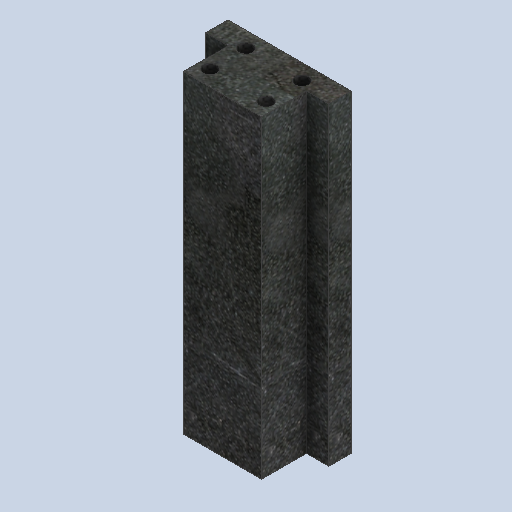
# Autodesk Inventor part: Fuhrung
Saved by Autodesk Inventor 2023.2 (Build 272271000, 271)
## iProperties
Created: 2023-02-07
Part Number: Fuhrung
Material: Steel
Document SubType Name: Modeling
Designer: Ayush
Density: 7.85 g/cm^3
Appearance: Plate
Author: Ayush
Autodesk Inventor part; units mm, degrees
ref_plane "YZ Plane" through (0, 0, 0) normal (1, 0, 0) x (0, 1, 0)
ref_plane "XZ Plane" through (0, 0, 0) normal (0, 1, 0) x (-1, 0, 0)
ref_plane "XY Plane" through (0, 0, 0) normal (0, 0, 1) x (1, 0, 0)
sketch "Sketch1" plane through (0, 0, 0) normal (0, 1, 0) x (-1, 0, 0)
  line L0 (17.5, 0) -> (-17.5, 0)
  line L1 (27.5, -30) -> (-27.5, -30)
  line L2 (27.5, -30) -> (27.5, -20)
  line L3 (27.5, -20) -> (17.5, -20)
  line L4 (-27.5, -30) -> (-27.5, -20)
  line L5 (-27.5, -20) -> (-17.5, -20)
  line L6 (17.5, -20) -> (17.5, 0)
  line L7 (-17.5, -20) -> (-17.5, 0)
  circle A0 centre (12.5, -23) radius 3
  circle A1 centre (-12.5, -23) radius 3
  circle A2 centre (-12.5, -7) radius 3
  circle A3 centre (12.5, -7) radius 3
  point P0 (0, 0)
  dimension "d2" = 35
  dimension "d8" = 55
  dimension "d9" = 10
  dimension "d10" = 10
  dimension "d11" = 6
  dimension "d12" = 6
  dimension "d13" = 6
  dimension "d14" = 6
  dimension "d17" = 7
  dimension "d18" = 16
  constraints: 16 end point, 4 centre point, 2 horizontal, 2 horizontal alignment, 2 perpendicular, 2 vertical, 2 vertical alignment, 1 parallel
  measures "d2" distance of L0.start L0.end
  measures "d8" distance of L1.start L1.end
  measures "d9" distance of L1.start L2.end
  measures "d10" distance of L1.end L4.end
  measures "d11" diameter of A0
  measures "d12" diameter of A1
  measures "d13" diameter of A2
  measures "d14" diameter of A3
  measures "d17" distance from line of A3.centre L0
  measures "d18" distance of A0.centre A3.centre
extrude "Extrusion1" add sketch "Sketch1" along normal blind 30
sketch "Sketch4" plane through (0, 0, 0) normal (0, -1, 0) x (1, 0, 0)
  line L0 (27.5, -20) -> (27.5, -30) projected
  line L1 (27.5, -30) -> (-27.5, -30) projected
  line L2 (27.5, -30) -> (-27.5, -30)
  line L3 (-27.5, -30) -> (-27.5, -20) projected
  line L4 (-27.5, -30) -> (-27.5, -20)
  line L5 (-27.5, -20) -> (-17.5, -20) projected
  line L6 (-27.5, -20) -> (-17.5, -20)
  line L7 (-17.5, -20) -> (-17.5, 0) projected
  line L8 (-17.5, -20) -> (-17.5, 0)
  line L9 (-17.5, 0) -> (17.5, 0) projected
  line L10 (-17.5, 0) -> (17.5, 0)
  line L11 (17.5, 0) -> (17.5, -20) projected
  line L12 (17.5, 0) -> (17.5, -20)
  line L13 (17.5, -20) -> (27.5, -20)
  line L14 (27.5, -20) -> (27.5, -30)
  point P0 (0, 0)
  constraints: 16 end point, 4 perpendicular, 3 collinear, 1 point on line
extrude "Extrusion3" add sketch "Sketch4" along normal blind 70
sketch "Sketch5" plane through (0, -70, 0) normal (0, -1, 0) x (1, 0, 0)
  line L0 (27.5, -30) -> (-27.5, -30) projected
  line L1 (27.5, -30) -> (-27.5, -30)
  line L2 (-27.5, -30) -> (-27.5, -20) projected
  line L3 (-27.5, -30) -> (-27.5, -20)
  line L4 (-27.5, -20) -> (-17.5, -20) projected
  line L5 (-27.5, -20) -> (-17.5, -20)
  line L6 (-17.5, -20) -> (-17.5, 0) projected
  line L7 (-17.5, -20) -> (-17.5, 0)
  line L8 (-17.5, 0) -> (17.5, 0)
  line L9 (17.5, 0) -> (17.5, -20) projected
  line L10 (17.5, 0) -> (17.5, -20)
  line L11 (17.5, -20) -> (27.5, -20) projected
  line L12 (17.5, -20) -> (27.5, -20)
  line L13 (27.5, -20) -> (27.5, -30) projected
  line L14 (27.5, -20) -> (27.5, -30)
  circle A0 centre (0, -8) radius 4
  circle A1 centre (10.5, -23) radius 4
  circle A2 centre (-10.5, -23) radius 4
  point P0 (0, 0)
  dimension "d25" = 8
  dimension "d26" = 8
  dimension "d27" = 8
  dimension "d28" = 10.5
  dimension "d29" = 10.5
  dimension "d30" = 8
  dimension "d31" = 15
  constraints: 16 end point, 6 collinear, 3 centre point, 1 horizontal, 1 horizontal alignment, 1 perpendicular
  measures "d25" diameter of A0
  measures "d26" diameter of A1
  measures "d27" diameter of A2
  measures "d28" horizontal distance of A2.centre A0.centre
  measures "d29" horizontal distance of A1.centre A0.centre
  measures "d30" distance from line of A0.centre L8
  measures "d31" vertical distance of A1.centre A0.centre
extrude "Extrusion4" add sketch "Sketch5" along normal blind 40
sketch "Sketch6" plane through (27.5, 30, -30) normal (0, 0, -1) x (-1, 0, 0)
  circle A0 centre (40, -105.0156) radius 3
  circle A1 centre (15, -105.0156) radius 3
  circle A2 centre (15, -60.0156) radius 3
  line L0 (55, -140) -> (0, -140) projected
  line L1 (27.5, 4.7422) -> (27.5, -229.8437)
  line L2 (55, -140) -> (55, 0) projected
  circle A3 centre (40, -60.0156) radius 3
  circle A4 centre (15, -15.0156) radius 3
  circle A5 centre (40, -15.0156) radius 3
  point P0 (27.5, -30)
  dimension "d35" = 6
  dimension "d38" = 6
  dimension "d39" = 6
  dimension "d42" = 45
  dimension "d43" = 27.5
  dimension "d44" = 12.5
  dimension "d53" = 6
  dimension "d54" = 6
  dimension "d55" = 6
  dimension "d56" = 45
  dimension "d57" = 45
  constraints: 6 centre point, 2 end point, 2 horizontal alignment, 2 vertical alignment, 1 coincident, 1 perpendicular
  measures "d35" diameter of A0
  measures "d38" diameter of A1
  measures "d39" diameter of A2
  measures "d42" distance of point (40, -60.016) A0.centre
  measures "d43" distance between parallel lines of L1 L2
  measures "d44" distance from line of point (40, -60.016) L1
  measures "d53" diameter of A3
  measures "d54" diameter of A4
  measures "d55" diameter of A5
  measures "d56" distance of A4.centre A2.centre
  measures "d57" distance of A5.centre point (40, -60.016)
hole "Hole1" at (-12.5, -75.0156, -30) at (12.5, -75.0156, -30) at (-12.5, -30.0156, -30) at (12.5, -30.0156, -30) at (12.5, 14.9844, -30) at (-12.5, 14.9844, -30) direction (0, 0, 1) diameter 6 depth 15 tip angle 118
body "Solid1"
